Autodesk Inventor part; units mm, degrees
(part 2 of 2)
sketch "Walls" plane through (0, 0, 0) normal (0, 0, -1) x (-1, 0, 0)
  circle A0 centre (92.5, -88.125) radius 2 projected
  circle A1 centre (48.3, 83.625) radius 1.55 projected
  circle A2 centre (-16.5, 83.625) radius 1.55 projected
  circle A3 centre (-80.1, 83.625) radius 1.55 projected
  circle A4 centre (-15.3, -1.621) radius 1.55 projected
  circle A5 centre (80.1, -26.621) radius 1.55 projected
  circle A6 centre (-48.3, -26.621) radius 1.55 projected
  circle A7 centre (-15.3, -26.621) radius 1.55 projected
  circle A8 centre (80.1, -1.621) radius 1.55 projected
  circle A9 centre (-48.3, -1.621) radius 1.55 projected
  circle A10 centre (-48.3, 58.625) radius 1.55 projected
  circle A11 centre (16.5, 58.625) radius 1.55 projected
  circle A12 centre (80.1, 58.625) radius 1.55 projected
  circle A13 centre (48.3, 58.625) radius 1.55 projected
  circle A14 centre (-16.5, 58.625) radius 1.55 projected
  circle A15 centre (-80.1, 58.625) radius 1.55 projected
  circle A16 centre (16.5, -1.621) radius 1.55 projected
  circle A17 centre (48.3, -26.621) radius 1.55 projected
  circle A18 centre (-80.1, -26.621) radius 1.55 projected
  circle A19 centre (16.5, -26.621) radius 1.55 projected
  circle A20 centre (48.3, -1.621) radius 1.55 projected
  circle A21 centre (-80.1, -1.621) radius 1.55 projected
  circle A22 centre (-48.3, 83.625) radius 1.55 projected
  circle A23 centre (16.5, 83.625) radius 1.55 projected
  circle A24 centre (80.1, 83.625) radius 1.55 projected
  arc A25 (-14.4, 61.625) -> (-10.35, 65.675) centre (-14.4, 65.675) ccw projected
  line L0 (-14.4, 61.625) -> (-18.6, 61.625) projected
  arc A26 (-22.65, 65.675) -> (-18.6, 61.625) centre (-18.6, 65.675) ccw projected
  line L1 (-22.65, 65.675) -> (-22.65, 79.375) projected
  arc A27 (-21.4, 80.625) -> (-22.65, 79.375) centre (-21.4, 79.375) ccw projected
  line L2 (-21.4, 80.625) -> (-11.6, 80.625) projected
  arc A28 (-10.35, 79.375) -> (-11.6, 80.625) centre (-11.6, 79.375) ccw projected
  line L3 (-10.35, 79.375) -> (-10.35, 65.675) projected
  line L4 (-69.055, 14.153) -> (-91.145, 14.153) projected
  line L5 (-91.145, 14.153) -> (-91.145, 43.101) projected
  line L6 (-91.145, 43.101) -> (-69.055, 43.101) projected
  line L7 (-69.055, 43.101) -> (-69.055, 14.153) projected
  line L8 (59.345, 43.101) -> (59.345, 14.153) projected
  line L9 (59.345, 14.153) -> (37.255, 14.153) projected
  line L10 (37.255, 14.153) -> (37.255, 43.101) projected
  line L11 (37.255, 43.101) -> (59.345, 43.101) projected
  arc A29 (18.6, -23.621) -> (22.65, -19.571) centre (18.6, -19.571) ccw projected
  line L12 (18.6, -23.621) -> (14.4, -23.621) projected
  arc A30 (10.35, -19.571) -> (14.4, -23.621) centre (14.4, -19.571) ccw projected
  line L13 (10.35, -19.571) -> (10.35, -5.871) projected
  arc A31 (11.6, -4.621) -> (10.35, -5.871) centre (11.6, -5.871) ccw projected
  line L14 (11.6, -4.621) -> (21.4, -4.621) projected
  arc A32 (22.65, -5.871) -> (21.4, -4.621) centre (21.4, -5.871) ccw projected
  line L15 (22.65, -5.871) -> (22.65, -19.571) projected
  line L16 (-69.055, -42.145) -> (-69.055, -71.093) projected
  line L17 (-69.055, -71.093) -> (-91.145, -71.093) projected
  line L18 (-91.145, -71.093) -> (-91.145, -42.145) projected
  line L19 (-91.145, -42.145) -> (-69.055, -42.145) projected
  line L20 (59.345, -42.145) -> (59.345, -71.093) projected
  line L21 (59.345, -71.093) -> (37.255, -71.093) projected
  line L22 (37.255, -71.093) -> (37.255, -42.145) projected
  line L23 (37.255, -42.145) -> (59.345, -42.145) projected
  line L24 (27.545, -42.145) -> (27.545, -71.093) projected
  line L25 (27.545, -71.093) -> (5.455, -71.093) projected
  line L26 (5.455, -71.093) -> (5.455, -42.145) projected
  line L27 (5.455, -42.145) -> (27.545, -42.145) projected
  arc A33 (-86.25, -19.571) -> (-82.2, -23.621) centre (-82.2, -19.571) ccw projected
  line L28 (-86.25, -19.571) -> (-86.25, -5.871) projected
  arc A34 (-85, -4.621) -> (-86.25, -5.871) centre (-85, -5.871) ccw projected
  line L29 (-85, -4.621) -> (-75.2, -4.621) projected
  arc A35 (-73.95, -5.871) -> (-75.2, -4.621) centre (-75.2, -5.871) ccw projected
  line L30 (-73.95, -5.871) -> (-73.95, -19.571) projected
  arc A36 (-78, -23.621) -> (-73.95, -19.571) centre (-78, -19.571) ccw projected
  line L31 (-78, -23.621) -> (-82.2, -23.621) projected
  arc A37 (50.4, -23.621) -> (54.45, -19.571) centre (50.4, -19.571) ccw projected
  line L32 (50.4, -23.621) -> (46.2, -23.621) projected
  arc A38 (42.15, -19.571) -> (46.2, -23.621) centre (46.2, -19.571) ccw projected
  line L33 (42.15, -19.571) -> (42.15, -5.871) projected
  arc A39 (43.4, -4.621) -> (42.15, -5.871) centre (43.4, -5.871) ccw projected
  line L34 (43.4, -4.621) -> (53.2, -4.621) projected
  arc A40 (54.45, -5.871) -> (53.2, -4.621) centre (53.2, -5.871) ccw projected
  line L35 (54.45, -5.871) -> (54.45, -19.571) projected
  line L36 (27.545, 43.101) -> (27.545, 14.153) projected
  line L37 (27.545, 14.153) -> (5.455, 14.153) projected
  line L38 (5.455, 14.153) -> (5.455, 43.101) projected
  line L39 (5.455, 43.101) -> (27.545, 43.101) projected
  arc A41 (82.2, 61.625) -> (86.25, 65.675) centre (82.2, 65.675) ccw projected
  line L40 (82.2, 61.625) -> (78, 61.625) projected
  arc A42 (73.95, 65.675) -> (78, 61.625) centre (78, 65.675) ccw projected
  line L41 (73.95, 65.675) -> (73.95, 79.375) projected
  arc A43 (75.2, 80.625) -> (73.95, 79.375) centre (75.2, 79.375) ccw projected
  line L42 (75.2, 80.625) -> (85, 80.625) projected
  arc A44 (86.25, 79.375) -> (85, 80.625) centre (85, 79.375) ccw projected
  line L43 (86.25, 79.375) -> (86.25, 65.675) projected
  arc A45 (-46.2, 61.625) -> (-42.15, 65.675) centre (-46.2, 65.675) ccw projected
  line L44 (-46.2, 61.625) -> (-50.4, 61.625) projected
  arc A46 (-54.45, 65.675) -> (-50.4, 61.625) centre (-50.4, 65.675) ccw projected
  line L45 (-54.45, 65.675) -> (-54.45, 79.375) projected
  arc A47 (-53.2, 80.625) -> (-54.45, 79.375) centre (-53.2, 79.375) ccw projected
  line L46 (-53.2, 80.625) -> (-43.4, 80.625) projected
  arc A48 (-42.15, 79.375) -> (-43.4, 80.625) centre (-43.4, 79.375) ccw projected
  line L47 (-42.15, 79.375) -> (-42.15, 65.675) projected
  arc A49 (18.6, 61.625) -> (22.65, 65.675) centre (18.6, 65.675) ccw projected
  line L48 (18.6, 61.625) -> (14.4, 61.625) projected
  arc A50 (10.35, 65.675) -> (14.4, 61.625) centre (14.4, 65.675) ccw projected
  line L49 (10.35, 65.675) -> (10.35, 79.375) projected
  arc A51 (11.6, 80.625) -> (10.35, 79.375) centre (11.6, 79.375) ccw projected
  line L50 (11.6, 80.625) -> (21.4, 80.625) projected
  arc A52 (22.65, 79.375) -> (21.4, 80.625) centre (21.4, 79.375) ccw projected
  line L51 (22.65, 79.375) -> (22.65, 65.675) projected
  line L52 (-37.255, 43.101) -> (-37.255, 14.153) projected
  line L53 (-37.255, 14.153) -> (-59.345, 14.153) projected
  line L54 (-59.345, 14.153) -> (-59.345, 43.101) projected
  line L55 (-59.345, 43.101) -> (-37.255, 43.101) projected
  line L56 (91.145, 43.101) -> (91.145, 14.153) projected
  line L57 (91.145, 14.153) -> (69.055, 14.153) projected
  line L58 (69.055, 14.153) -> (69.055, 43.101) projected
  line L59 (69.055, 43.101) -> (91.145, 43.101) projected
  arc A53 (-13.2, -23.621) -> (-9.15, -19.571) centre (-13.2, -19.571) ccw projected
  line L60 (-13.2, -23.621) -> (-17.4, -23.621) projected
  arc A54 (-21.45, -19.571) -> (-17.4, -23.621) centre (-17.4, -19.571) ccw projected
  line L61 (-21.45, -19.571) -> (-21.45, -5.871) projected
  arc A55 (-20.2, -4.621) -> (-21.45, -5.871) centre (-20.2, -5.871) ccw projected
  line L62 (-20.2, -4.621) -> (-10.4, -4.621) projected
  arc A56 (-9.15, -5.871) -> (-10.4, -4.621) centre (-10.4, -5.871) ccw projected
  line L63 (-9.15, -5.871) -> (-9.15, -19.571) projected
  line L64 (-37.255, -42.145) -> (-37.255, -71.093) projected
  line L65 (-37.255, -71.093) -> (-59.345, -71.093) projected
  line L66 (-59.345, -71.093) -> (-59.345, -42.145) projected
  line L67 (-59.345, -42.145) -> (-37.255, -42.145) projected
  line L68 (91.145, -42.145) -> (91.145, -71.093) projected
  line L69 (91.145, -71.093) -> (69.055, -71.093) projected
  line L70 (69.055, -71.093) -> (69.055, -42.145) projected
  line L71 (69.055, -42.145) -> (91.145, -42.145) projected
  line L72 (-4.255, -42.145) -> (-4.255, -71.093) projected
  line L73 (-4.255, -71.093) -> (-26.345, -71.093) projected
  line L74 (-26.345, -71.093) -> (-26.345, -42.145) projected
  line L75 (-26.345, -42.145) -> (-4.255, -42.145) projected
  arc A57 (-46.2, -23.621) -> (-42.15, -19.571) centre (-46.2, -19.571) ccw projected
  line L76 (-46.2, -23.621) -> (-50.4, -23.621) projected
  arc A58 (-54.45, -19.571) -> (-50.4, -23.621) centre (-50.4, -19.571) ccw projected
  line L77 (-54.45, -19.571) -> (-54.45, -5.871) projected
  arc A59 (-53.2, -4.621) -> (-54.45, -5.871) centre (-53.2, -5.871) ccw projected
  line L78 (-53.2, -4.621) -> (-43.4, -4.621) projected
  arc A60 (-42.15, -5.871) -> (-43.4, -4.621) centre (-43.4, -5.871) ccw projected
  line L79 (-42.15, -5.871) -> (-42.15, -19.571) projected
  arc A61 (82.2, -23.621) -> (86.25, -19.571) centre (82.2, -19.571) ccw projected
  line L80 (82.2, -23.621) -> (78, -23.621) projected
  arc A62 (73.95, -19.571) -> (78, -23.621) centre (78, -19.571) ccw projected
  line L81 (73.95, -19.571) -> (73.95, -5.871) projected
  arc A63 (75.2, -4.621) -> (73.95, -5.871) centre (75.2, -5.871) ccw projected
  line L82 (75.2, -4.621) -> (85, -4.621) projected
  arc A64 (86.25, -5.871) -> (85, -4.621) centre (85, -5.871) ccw projected
  line L83 (86.25, -5.871) -> (86.25, -19.571) projected
  line L84 (-5.455, 43.101) -> (-5.455, 14.153) projected
  line L85 (-5.455, 14.153) -> (-27.545, 14.153) projected
  line L86 (-27.545, 14.153) -> (-27.545, 43.101) projected
  line L87 (-27.545, 43.101) -> (-5.455, 43.101) projected
  arc A65 (50.4, 61.625) -> (54.45, 65.675) centre (50.4, 65.675) ccw projected
  line L88 (50.4, 61.625) -> (46.2, 61.625) projected
  arc A66 (42.15, 65.675) -> (46.2, 61.625) centre (46.2, 65.675) ccw projected
  line L89 (42.15, 65.675) -> (42.15, 79.375) projected
  arc A67 (43.4, 80.625) -> (42.15, 79.375) centre (43.4, 79.375) ccw projected
  line L90 (43.4, 80.625) -> (53.2, 80.625) projected
  arc A68 (54.45, 79.375) -> (53.2, 80.625) centre (53.2, 79.375) ccw projected
  line L91 (54.45, 79.375) -> (54.45, 65.675) projected
  arc A69 (-86.25, 65.675) -> (-82.2, 61.625) centre (-82.2, 65.675) ccw projected
  line L92 (-86.25, 65.675) -> (-86.25, 79.375) projected
  arc A70 (-85, 80.625) -> (-86.25, 79.375) centre (-85, 79.375) ccw projected
  line L93 (-85, 80.625) -> (-75.2, 80.625) projected
  arc A71 (-73.95, 79.375) -> (-75.2, 80.625) centre (-75.2, 79.375) ccw projected
  line L94 (-73.95, 79.375) -> (-73.95, 65.675) projected
  arc A72 (-78, 61.625) -> (-73.95, 65.675) centre (-78, 65.675) ccw projected
  line L95 (-78, 61.625) -> (-82.2, 61.625) projected
  circle A73 centre (92.5, -88.125) radius 2 projected
  circle A74 centre (-92.5, 88.125) radius 2 projected
  circle A75 centre (-92.5, -88.125) radius 2 projected
  circle A76 centre (92.5, 88.125) radius 2 projected
  arc A77 (93.6716, 96.9534) -> (90.8431, 98.125) centre (90.8431, 94.125) ccw projected
  line L96 (-90.8431, 98.125) -> (90.8431, 98.125) projected
  arc A78 (-90.8431, 98.125) -> (-93.6716, 96.9534) centre (-90.8431, 94.125) ccw projected
  line L97 (-101.3284, 89.2966) -> (-93.6716, 96.9534) projected
  arc A79 (-101.3284, 89.2966) -> (-102.5, 86.4681) centre (-98.5, 86.4681) ccw projected
  line L98 (-102.5, -86.4681) -> (-102.5, 86.4681) projected
  arc A80 (-102.5, -86.4681) -> (-101.3284, -89.2966) centre (-98.5, -86.4681) ccw projected
  line L99 (-93.6716, -96.9534) -> (-101.3284, -89.2966) projected
  arc A81 (-93.6716, -96.9534) -> (-90.8431, -98.125) centre (-90.8431, -94.125) ccw projected
  line L100 (90.8431, -98.125) -> (-90.8431, -98.125) projected
  arc A82 (90.8431, -98.125) -> (93.6716, -96.9534) centre (90.8431, -94.125) ccw projected
  line L101 (101.3284, -89.2966) -> (93.6716, -96.9534) projected
  arc A83 (101.3284, -89.2966) -> (102.5, -86.4681) centre (98.5, -86.4681) ccw projected
  line L102 (102.5, 86.4681) -> (102.5, -86.4681) projected
  arc A84 (102.5, 86.4681) -> (101.3284, 89.2966) centre (98.5, 86.4681) ccw projected
  line L103 (93.6716, 96.9534) -> (101.3284, 89.2966) projected
  circle A85 centre (-11, -88.625) radius 3.2 projected
  circle A86 centre (11, -88.625) radius 3.2 projected
  circle A87 centre (92.5, -88.125) radius 2 projected
  circle A88 centre (92.5, -88.125) radius 4
  circle A89 centre (92.5, 88.125) radius 2 projected
  circle A90 centre (92.5, 88.125) radius 4
  circle A91 centre (-92.5, 88.125) radius 2 projected
  circle A92 centre (-92.5, 88.125) radius 4
  circle A93 centre (-92.5, -88.125) radius 2 projected
  circle A94 centre (-92.5, -88.125) radius 4
  arc A95 (99.9142, -87.8824) -> (100.5, -86.4681) centre (98.5, -86.4681) ccw
  line L104 (99.9142, -87.8824) -> (92.2574, -95.5392)
  arc A96 (90.8431, -96.125) -> (92.2574, -95.5392) centre (90.8431, -94.125) ccw
  line L105 (90.8431, -96.125) -> (-90.8431, -96.125)
  arc A97 (-92.2574, -95.5392) -> (-90.8431, -96.125) centre (-90.8431, -94.125) ccw
  line L106 (-92.2574, -95.5392) -> (-99.9142, -87.8824)
  arc A98 (-100.5, -86.4681) -> (-99.9142, -87.8824) centre (-98.5, -86.4681) ccw
  line L107 (-100.5, -86.4681) -> (-100.5, 86.4681)
  arc A99 (-99.9142, 87.8824) -> (-100.5, 86.4681) centre (-98.5, 86.4681) ccw
  line L108 (-99.9142, 87.8824) -> (-92.2574, 95.5392)
  arc A100 (-90.8431, 96.125) -> (-92.2574, 95.5392) centre (-90.8431, 94.125) ccw
  line L109 (-90.8431, 96.125) -> (90.8431, 96.125)
  arc A101 (92.2574, 95.5392) -> (90.8431, 96.125) centre (90.8431, 94.125) ccw
  line L110 (92.2574, 95.5392) -> (99.9142, 87.8824)
  arc A102 (100.5, 86.4681) -> (99.9142, 87.8824) centre (98.5, 86.4681) ccw
  line L111 (100.5, 86.4681) -> (100.5, -86.4681)
  point P0 (0, 0)
  dimension "d92" = 8
  dimension "d93" = 8
  dimension "d94" = 8
  dimension "d95" = 8
  dimension "d96" = 2
  constraints: 16 end point, 16 point on circle, 12 centre point, 4 coincident, 15 other
  measures "d92" diameter of A88
  measures "d93" diameter of A90
  measures "d94" diameter of A92
  measures "d95" diameter of A94
  measures "d96" distance between parallel lines of L102 L111
extrude "WallsFeature" add sketch "Walls" along normal blind 10 contours L103 A84 L102 A83 L101 A82 L100 A81 L99 A80 L98 A79 L97 A78 L96 A77 | A88 | A90 | A92 | A94
sketch "Fills" plane through (0, 0, -10) normal (0, 0, -1) x (-1, 0, 0)
  line L0 (101.3284, 89.2966) -> (93.6716, 96.9534) projected
  arc A0 (93.6716, 96.9534) -> (90.8431, 98.125) centre (90.8431, 94.125) ccw projected
  line L1 (90.8431, 98.125) -> (-90.8431, 98.125) projected
  arc A1 (-90.8431, 98.125) -> (-93.6716, 96.9534) centre (-90.8431, 94.125) ccw projected
  line L2 (-93.6716, 96.9534) -> (-101.3284, 89.2966) projected
  arc A2 (-101.3284, 89.2966) -> (-102.5, 86.4681) centre (-98.5, 86.4681) ccw projected
  line L3 (-102.5, 86.4681) -> (-102.5, -86.4681) projected
  arc A3 (-102.5, -86.4681) -> (-101.3284, -89.2966) centre (-98.5, -86.4681) ccw projected
  line L4 (-101.3284, -89.2966) -> (-93.6716, -96.9534) projected
  arc A4 (-93.6716, -96.9534) -> (-90.8431, -98.125) centre (-90.8431, -94.125) ccw projected
  line L5 (-90.8431, -98.125) -> (90.8431, -98.125) projected
  arc A5 (90.8431, -98.125) -> (93.6716, -96.9534) centre (90.8431, -94.125) ccw projected
  line L6 (93.6716, -96.9534) -> (101.3284, -89.2966) projected
  arc A6 (101.3284, -89.2966) -> (102.5, -86.4681) centre (98.5, -86.4681) ccw projected
  line L7 (102.5, -86.4681) -> (102.5, 86.4681) projected
  arc A7 (102.5, 86.4681) -> (101.3284, 89.2966) centre (98.5, 86.4681) ccw projected
  line L8 (90.8431, -96.125) -> (-90.8431, -96.125) projected
  arc A8 (-92.2574, -95.5392) -> (-90.8431, -96.125) centre (-90.8431, -94.125) ccw projected
  line L9 (-92.2574, -95.5392) -> (-99.9142, -87.8824) projected
  arc A9 (-100.5, -86.4681) -> (-99.9142, -87.8824) centre (-98.5, -86.4681) ccw projected
  line L10 (-100.5, -86.4681) -> (-100.5, 86.4681) projected
  arc A10 (-99.9142, 87.8824) -> (-100.5, 86.4681) centre (-98.5, 86.4681) ccw projected
  line L11 (-99.9142, 87.8824) -> (-92.2574, 95.5392) projected
  arc A11 (-90.8431, 96.125) -> (-92.2574, 95.5392) centre (-90.8431, 94.125) ccw projected
  line L12 (-90.8431, 96.125) -> (90.8431, 96.125) projected
  arc A12 (92.2574, 95.5392) -> (90.8431, 96.125) centre (90.8431, 94.125) ccw projected
  line L13 (92.2574, 95.5392) -> (99.9142, 87.8824) projected
  arc A13 (100.5, 86.4681) -> (99.9142, 87.8824) centre (98.5, 86.4681) ccw projected
  line L14 (100.5, 86.4681) -> (100.5, -86.4681) projected
  arc A14 (99.9142, -87.8824) -> (100.5, -86.4681) centre (98.5, -86.4681) ccw projected
  line L15 (99.9142, -87.8824) -> (92.2574, -95.5392) projected
  arc A15 (90.8431, -96.125) -> (92.2574, -95.5392) centre (90.8431, -94.125) ccw projected
  circle A16 centre (92.5, -88.125) radius 4 projected
  circle A17 centre (92.5, -88.125) radius 2 projected
  circle A18 centre (-92.5, -88.125) radius 4 projected
  circle A19 centre (-92.5, -88.125) radius 2 projected
  circle A20 centre (-92.5, 88.125) radius 4 projected
  circle A21 centre (-92.5, 88.125) radius 2 projected
  circle A22 centre (92.5, 88.125) radius 4 projected
  circle A23 centre (92.5, 88.125) radius 2 projected
  line L16 (97.5, -93.125) -> (92.5, -88.125) construction
  line L17 (96.4393, -94.1857) -> (91.4393, -89.1857)
  line L18 (98.5607, -92.0643) -> (93.5607, -87.0643)
  line L19 (143.8938, 0) -> (-143.8938, 0) projected
  line L20 (0, -137.7688) -> (0, 137.7688) projected
  line L21 (-96.4393, -94.1857) -> (-91.4393, -89.1857)
  line L22 (-98.5607, -92.0643) -> (-93.5607, -87.0643)
  line L23 (96.4393, 94.1857) -> (91.4393, 89.1857)
  line L24 (98.5607, 92.0643) -> (93.5607, 87.0643)
  line L25 (-98.5607, 92.0643) -> (-93.5607, 87.0643)
  line L26 (-96.4393, 94.1857) -> (-91.4393, 89.1857)
  point P0 (0, 0)
  point P1 (95.0251, 92.7714)
  point P2 (94.0614, 91.8077)
  point P3 (96.1827, 89.6864)
  point P4 (97.1464, 90.6501)
  point P5 (-97.1464, 90.6501)
  point P6 (-96.1827, 89.6864)
  point P7 (-94.0614, 91.8077)
  point P8 (-95.0251, 92.7714)
  point P9 (-95.0251, -92.7714)
  point P10 (-94.0614, -91.8077)
  point P11 (-96.1827, -89.6864)
  point P12 (-97.1464, -90.6501)
  point P13 (97.1464, -90.6501)
  point P14 (96.1827, -89.6864)
  point P15 (94.0614, -91.8077)
  point P16 (95.0251, -92.7714)
  dimension "d99" = 1.5
  dimension "d100" = 1.5
  constraints: 18 end point, 12 symmetric about line, 2 parallel, 1 midpoint
  measures "d99" distance between parallel lines of L16 L17
  measures "d100" distance between parallel lines of L16 L18
extrude "FillsFeature" add sketch "Fills" against normal up to surface (10 mm away) contours L24 A22 L23 L13 | L15 L17 A16 L18 | L22 A18 L21 L9 | L11 L26 A20 L25
equation "\"d6\" = d5"
equation "\"d15\" = d5"
equation "\"d34\" = d33"
body "Solid1"
